Autodesk Fusion 360 part; units mm, degrees
note: some values were not read from the file. Chosen so that the rebuilt part matches the saved one: which bodies a step acts on.
(part 2 of 3)
sketch "DJ - Baxley - Dog Door (1)" plane through (0, 0, 0) normal (0, 1, 0) x (1, 0, 0)
  circle A0 through (-4.6949, -282.6663, -6.35) (-15.4673, -288.8858, -6.35) (-15.4673, -276.4469, -6.35)
  circle A1 through (-14.4863, -519.0473, -6.35) (-25.2588, -525.2667, -6.35) (-25.2588, -512.8278, -6.35)
  circle A2 through (-145.7196, -224.274, -6.35) (-156.4921, -230.4934, -6.35) (-156.4921, -218.0545, -6.35)
  circle A3 through (-70.3115, -135.2797, -6.35) (-81.084, -141.4992, -6.35) (-81.084, -129.0602, -6.35)
  circle A4 through (-80.103, -371.6606, -6.35) (-90.8754, -377.8801, -6.35) (-90.8754, -365.4411, -6.35)
  circle A5 through (60.9218, -430.053, -6.35) (50.1494, -436.2725, -6.35) (50.1494, -423.8335, -6.35)
  circle A6 through (51.1304, -666.4339, -6.35) (40.3579, -672.6534, -6.35) (40.3579, -660.2144, -6.35)
  circle A7 through (126.5385, -577.4396, -6.35) (115.766, -583.6591, -6.35) (115.766, -571.2202, -6.35)
  arc A8 through (0.0572, -283.1665, -6.35) (0.0572, -283.1665, -6.35) (0.0572, -283.1665, -6.35)
  arc A9 through (-65.5595, -135.7798, -6.35) (-65.5595, -135.7798, -6.35) (-65.5595, -135.7798, -6.35)
  arc A10 through (-9.7343, -519.5474, -6.35) (-9.7343, -519.5474, -6.35) (-9.7343, -519.5474, -6.35)
  arc A11 through (55.8824, -666.9341, -6.35) (55.8824, -666.9341, -6.35) (55.8824, -666.9341, -6.35)
  arc A12 through (65.6738, -430.5531, -6.35) (65.6738, -430.5531, -6.35) (65.6738, -430.5531, -6.35)
  arc A13 through (131.2905, -577.9398, -6.35) (131.2905, -577.9398, -6.35) (131.2905, -577.9398, -6.35)
  arc A14 through (-140.9676, -224.7741, -6.35) (-140.9676, -224.7741, -6.35) (-140.9676, -224.7741, -6.35)
  arc A15 through (-75.351, -372.1608, -6.35) (-75.351, -372.1608, -6.35) (-75.351, -372.1608, -6.35)
  circle A16 through (11.5572, -288.9047, -6.35) (0.7848, -295.1242, -6.35) (0.7848, -282.6852, -6.35)
  circle A17 through (1.7658, -525.2856, -6.35) (-9.0067, -531.5051, -6.35) (-9.0067, -519.0661, -6.35)
  circle A18 through (142.7906, -583.678, -6.35) (132.0181, -589.8975, -6.35) (132.0181, -577.4585, -6.35)
  circle A19 through (67.3825, -672.6723, -6.35) (56.61, -678.8917, -6.35) (56.61, -666.4528, -6.35)
  circle A20 through (77.1739, -436.2913, -6.35) (66.4015, -442.5108, -6.35) (66.4015, -430.0719, -6.35)
  circle A21 through (-129.4675, -230.5123, -6.35) (-140.24, -236.7318, -6.35) (-140.24, -224.2928, -6.35)
  circle A22 through (-54.0594, -141.518, -6.35) (-64.8319, -147.7375, -6.35) (-64.8319, -135.2986, -6.35)
  circle A23 through (-63.8509, -377.899, -6.35) (-74.6233, -384.1184, -6.35) (-74.6233, -371.6795, -6.35)
  circle A24 through (-46.9836, -370.3901, -6.35) (-57.756, -376.6096, -6.35) (-57.756, -364.1706, -6.35)
  circle A25 through (94.0412, -428.7825, -6.35) (83.2687, -435.0019, -6.35) (83.2687, -422.563, -6.35)
  circle A26 through (28.4245, -281.3958, -6.35) (17.6521, -287.6153, -6.35) (17.6521, -275.1763, -6.35)
  circle A27 through (84.2497, -665.1634, -6.35) (73.4773, -671.3829, -6.35) (73.4773, -658.9439, -6.35)
  circle A28 through (159.6579, -576.1691, -6.35) (148.8854, -582.3886, -6.35) (148.8854, -569.9496, -6.35)
  circle A29 through (18.6331, -517.7768, -6.35) (7.8606, -523.9962, -6.35) (7.8606, -511.5573, -6.35)
  circle A30 through (-37.1921, -134.0092, -6.35) (-47.9646, -140.2286, -6.35) (-47.9646, -127.7897, -6.35)
  circle A31 through (-112.6003, -223.0034, -6.35) (-123.3727, -229.2229, -6.35) (-123.3727, -216.784, -6.35)
  arc A32 through (11.5363, -288.3559, -6.35) (11.5363, -288.3559, -6.35) (11.5363, -288.3559, -6.35)
  arc A33 through (67.3615, -672.1235, -6.35) (67.3615, -672.1235, -6.35) (67.3615, -672.1235, -6.35)
  arc A34 through (77.1529, -435.7426, -6.35) (77.1529, -435.7426, -6.35) (77.1529, -435.7426, -6.35)
  arc A35 through (1.7448, -524.7369, -6.35) (1.7448, -524.7369, -6.35) (1.7448, -524.7369, -6.35)
  arc A36 through (142.7696, -583.1292, -6.35) (142.7696, -583.1292, -6.35) (142.7696, -583.1292, -6.35)
  arc A37 through (-63.8719, -377.3502, -6.35) (-63.8719, -377.3502, -6.35) (-63.8719, -377.3502, -6.35)
  arc A38 through (-129.4885, -229.9636, -6.35) (-129.4885, -229.9636, -6.35) (-129.4885, -229.9636, -6.35)
  arc A39 through (-54.0804, -140.9693, -6.35) (-54.0804, -140.9693, -6.35) (-54.0804, -140.9693, -6.35)
  circle A40 through (-40.7457, -354.1386, -6.35) (-51.5195, -360.3588, -6.35) (-51.5195, -347.9183, -6.35)
  circle A41 through (100.2791, -412.531, -6.35) (89.5053, -418.7512, -6.35) (89.5053, -406.3107, -6.35)
  circle A42 through (90.4876, -648.9119, -6.35) (79.7139, -655.1322, -6.35) (79.7139, -642.6916, -6.35)
  circle A43 through (34.6624, -265.1443, -6.35) (23.8886, -271.3646, -6.35) (23.8886, -258.9241, -6.35)
  circle A44 through (165.8958, -559.9176, -6.35) (155.122, -566.1379, -6.35) (155.122, -553.6974, -6.35)
  circle A45 through (24.871, -501.5252, -6.35) (14.0972, -507.7455, -6.35) (14.0972, -495.305, -6.35)
  circle A46 through (-106.3624, -206.7519, -6.35) (-117.1361, -212.9722, -6.35) (-117.1361, -200.5317, -6.35)
  circle A47 through (-30.9542, -117.7577, -6.35) (-41.728, -123.9779, -6.35) (-41.728, -111.5374, -6.35)
  arc A48 through (15.5928, -264.4328, -6.35) (15.6784, -265.1583, -6.35) (15.7364, -265.8867, -6.35)
  arc A49 through (51.9111, -657.7321, -6.35) (51.4996, -657.2579, -6.35) (51.0651, -656.8045, -6.35)
  arc A50 through (-11.9619, -270.2306, -6.35) (-17.8102, -266.2727, -6.35) (-19.7177, -259.4735, -6.35)
  arc A51 through (123.743, -544.5786, -6.35) (128.4893, -543.0332, -6.35) (132.5528, -540.1342, -6.35)
  arc A52 through (58.4262, -627.8801, -6.35) (72.1411, -628.2628, -6.35) (73.2112, -641.9413, -6.35)
  arc A53 through (71.5616, -649.6543, -6.35) (64.5815, -660.6144, -6.35) (51.9111, -657.7321, -6.35)
  arc A54 through (-4.7601, -273.037, -6.35) (-7.0021, -271.4358, -6.35) (-9.622, -270.5836, -6.35)
  arc A55 through (-59.6718, -354.8809, -6.35) (-66.6518, -365.8411, -6.35) (-79.3222, -362.9588, -6.35)
  arc A56 through (-95.1258, -348.4678, -6.35) (-92.29, -342.1526, -6.35) (-86.0885, -339.0761, -6.35)
  arc A57 through (-72.8072, -333.1068, -6.35) (-59.0922, -333.4895, -6.35) (-58.0221, -347.168, -6.35)
  arc A58 through (-17.2817, -486.1862, -6.35) (-12.5354, -484.6408, -6.35) (-8.472, -481.7418, -6.35)
  arc A59 through (120.553, -544.8551, -6.35) (122.1526, -544.7694, -6.35) (123.743, -544.5786, -6.35)
  arc A60 through (111.5156, -554.2468, -6.35) (114.3515, -547.9316, -6.35) (120.553, -544.8551, -6.35)
  arc A61 through (-79.3222, -362.9588, -6.35) (-79.7338, -362.4846, -6.35) (-80.1682, -362.0312, -6.35)
  arc A62 through (15.7364, -265.8867, -6.35) (8.7563, -276.8468, -6.35) (-3.9141, -273.9645, -6.35)
  arc A63 through (-19.7177, -259.4735, -6.35) (-16.8819, -253.1583, -6.35) (-10.6804, -250.0818, -6.35)
  arc A64 through (66.9361, -392.7476, -6.35) (67.5597, -392.1057, -6.35) (68.2176, -391.4992, -6.35)
  arc A65 through (-19.4134, -506.9645, -6.35) (-20.5908, -506.8371, -6.35) (-21.7533, -506.6116, -6.35)
  arc A66 through (45.899, -406.8602, -6.35) (48.7348, -400.545, -6.35) (54.9363, -397.4685, -6.35)
  arc A67 through (81.2094, -411.8194, -6.35) (81.2951, -412.545, -6.35) (81.353, -413.2733, -6.35)
  arc A68 through (-21.7533, -506.6116, -6.35) (-27.6017, -502.6537, -6.35) (-29.5091, -495.8545, -6.35)
  arc A69 through (5.8013, -500.8137, -6.35) (5.887, -501.5393, -6.35) (5.9449, -502.2676, -6.35)
  arc A70 through (81.353, -413.2733, -6.35) (74.373, -424.2335, -6.35) (61.7026, -421.3511, -6.35)
  arc A71 through (73.2112, -641.9413, -6.35) (71.7329, -644.9042, -6.35) (71.418, -648.2004, -6.35)
  arc A72 through (-85.0301, -359.5779, -6.35) (-86.2074, -359.4504, -6.35) (-87.37, -359.2249, -6.35)
  arc A73 through (146.9697, -560.66, -6.35) (139.9896, -571.6201, -6.35) (127.3193, -568.7378, -6.35)
  arc A74 through (-7.1905, -480.4935, -6.35) (6.5245, -480.8762, -6.35) (7.5945, -494.5547, -6.35)
  arc A75 through (146.8261, -559.2061, -6.35) (146.9118, -559.9317, -6.35) (146.9697, -560.66, -6.35)
  arc A76 through (17.386, -258.1737, -6.35) (15.9077, -261.1366, -6.35) (15.5928, -264.4328, -6.35)
  arc A77 through (-8.472, -481.7418, -6.35) (-7.8484, -481.1, -6.35) (-7.1905, -480.4935, -6.35)
  arc A78 through (36.1075, -643.2411, -6.35) (38.9434, -636.9259, -6.35) (45.1449, -633.8494, -6.35)
  arc A79 through (-82.8984, -338.7996, -6.35) (-78.1521, -337.2542, -6.35) (-74.0887, -334.3552, -6.35)
  arc A80 through (55.9947, -417.9702, -6.35) (54.8173, -417.8428, -6.35) (53.6548, -417.6173, -6.35)
  arc A81 through (60.8566, -420.4236, -6.35) (58.6146, -418.8224, -6.35) (55.9947, -417.9702, -6.35)
  arc A82 through (71.418, -648.2004, -6.35) (71.5036, -648.9259, -6.35) (71.5616, -649.6543, -6.35)
  arc A83 through (51.0651, -656.8045, -6.35) (48.8231, -655.2034, -6.35) (46.2032, -654.3512, -6.35)
  arc A84 through (133.8343, -538.8858, -6.35) (147.5492, -539.2685, -6.35) (148.6193, -552.9471, -6.35)
  arc A85 through (-80.1682, -362.0312, -6.35) (-82.4102, -360.4301, -6.35) (-85.0301, -359.5779, -6.35)
  arc A86 through (132.5528, -540.1342, -6.35) (133.1764, -539.4924, -6.35) (133.8343, -538.8858, -6.35)
  arc A87 through (-13.7055, -510.3454, -6.35) (-14.1171, -509.8712, -6.35) (-14.5516, -509.4179, -6.35)
  arc A88 through (-14.5516, -509.4179, -6.35) (-16.7935, -507.8167, -6.35) (-19.4134, -506.9645, -6.35)
  arc A89 through (-74.0887, -334.3552, -6.35) (-73.4651, -333.7134, -6.35) (-72.8072, -333.1068, -6.35)
  arc A90 through (53.6548, -417.6173, -6.35) (47.8064, -413.6594, -6.35) (45.899, -406.8602, -6.35)
  arc A91 through (61.7026, -421.3511, -6.35) (61.291, -420.8769, -6.35) (60.8566, -420.4236, -6.35)
  arc A92 through (-59.8154, -353.4271, -6.35) (-59.7297, -354.1526, -6.35) (-59.6718, -354.8809, -6.35)
  arc A93 through (83.0027, -405.5604, -6.35) (81.5244, -408.5233, -6.35) (81.2094, -411.8194, -6.35)
  arc A94 through (43.8633, -653.9982, -6.35) (38.015, -650.0403, -6.35) (36.1075, -643.2411, -6.35)
  arc A95 through (68.2176, -391.4992, -6.35) (81.9326, -391.8819, -6.35) (83.0027, -405.5604, -6.35)
  arc A96 through (-29.5091, -495.8545, -6.35) (-26.6733, -489.5393, -6.35) (-20.4718, -486.4628, -6.35)
  arc A97 through (121.6114, -565.3569, -6.35) (120.434, -565.2294, -6.35) (119.2714, -565.0039, -6.35)
  arc A98 through (126.4732, -567.8103, -6.35) (124.2313, -566.2091, -6.35) (121.6114, -565.3569, -6.35)
  arc A99 through (-9.622, -270.5836, -6.35) (-10.7993, -270.4561, -6.35) (-11.9619, -270.2306, -6.35)
  arc A100 through (45.1449, -633.8494, -6.35) (46.7444, -633.7637, -6.35) (48.3349, -633.5729, -6.35)
  arc A101 through (148.6193, -552.9471, -6.35) (147.1411, -555.9099, -6.35) (146.8261, -559.2061, -6.35)
  arc A102 through (-7.4903, -249.8053, -6.35) (-2.744, -248.2599, -6.35) (1.3195, -245.3609, -6.35)
  arc A103 through (58.1264, -397.1919, -6.35) (62.8727, -395.6465, -6.35) (66.9361, -392.7476, -6.35)
  arc A104 through (48.3349, -633.5729, -6.35) (53.0812, -632.0275, -6.35) (57.1447, -629.1285, -6.35)
  arc A105 through (119.2714, -565.0039, -6.35) (113.4231, -561.0461, -6.35) (111.5156, -554.2468, -6.35)
  arc A106 through (7.5945, -494.5547, -6.35) (6.1163, -497.5176, -6.35) (5.8013, -500.8137, -6.35)
  arc A107 through (-20.4718, -486.4628, -6.35) (-18.8722, -486.377, -6.35) (-17.2817, -486.1862, -6.35)
  arc A108 through (-87.37, -359.2249, -6.35) (-93.2184, -355.267, -6.35) (-95.1258, -348.4678, -6.35)
  arc A109 through (-49.8803, -118.5, -6.35) (-56.8604, -129.4602, -6.35) (-69.5307, -126.5778, -6.35)
  arc A110 through (-150.6468, -212.1912, -6.35) (-151.8241, -212.0638, -6.35) (-152.9867, -211.8383, -6.35)
  arc A111 through (-85.3344, -112.0869, -6.35) (-82.4985, -105.7717, -6.35) (-76.297, -102.6952, -6.35)
  arc A112 through (1.3195, -245.3609, -6.35) (1.943, -244.7191, -6.35) (2.6009, -244.1125, -6.35)
  arc A113 through (-10.6804, -250.0818, -6.35) (-9.0808, -249.9961, -6.35) (-7.4903, -249.8053, -6.35)
  arc A114 through (-152.9867, -211.8383, -6.35) (-158.835, -207.8804, -6.35) (-160.7425, -201.0812, -6.35)
  arc A115 through (2.6009, -244.1125, -6.35) (16.3159, -244.4952, -6.35) (17.386, -258.1737, -6.35)
  arc A116 through (-160.7425, -201.0812, -6.35) (-157.9066, -194.766, -6.35) (-151.7051, -191.6894, -6.35)
  arc A117 through (54.9363, -397.4685, -6.35) (56.5359, -397.3827, -6.35) (58.1264, -397.1919, -6.35)
  arc A118 through (-64.2972, -97.9742, -6.35) (-63.6736, -97.3324, -6.35) (-63.0157, -96.7259, -6.35)
  arc A119 through (-63.0157, -96.7259, -6.35) (-49.3008, -97.1086, -6.35) (-48.2307, -110.7871, -6.35)
  arc A120 through (-77.5786, -122.844, -6.35) (-83.4269, -118.8861, -6.35) (-85.3344, -112.0869, -6.35)
  arc A121 through (5.9449, -502.2676, -6.35) (-1.0352, -513.2278, -6.35) (-13.7055, -510.3454, -6.35)
  arc A122 through (-151.7051, -191.6894, -6.35) (-150.1056, -191.6037, -6.35) (-148.5151, -191.4129, -6.35)
  arc A123 through (-69.5307, -126.5778, -6.35) (-69.9423, -126.1036, -6.35) (-70.3768, -125.6503, -6.35)
  arc A124 through (-125.2884, -207.4943, -6.35) (-132.2685, -218.4544, -6.35) (-144.9389, -215.5721, -6.35)
  arc A125 through (-125.432, -206.0404, -6.35) (-125.3464, -206.766, -6.35) (-125.2884, -207.4943, -6.35)
  arc A126 through (-73.107, -102.4186, -6.35) (-68.3607, -100.8732, -6.35) (-64.2972, -97.9742, -6.35)
  arc A127 through (-139.7053, -186.9685, -6.35) (-139.0818, -186.3267, -6.35) (-138.4238, -185.7202, -6.35)
  arc A128 through (127.3193, -568.7378, -6.35) (126.9077, -568.2636, -6.35) (126.4732, -567.8103, -6.35)
  arc A129 through (-58.0221, -347.168, -6.35) (-59.5004, -350.1309, -6.35) (-59.8154, -353.4271, -6.35)
  arc A130 through (-138.4238, -185.7202, -6.35) (-124.7089, -186.1029, -6.35) (-123.6388, -199.7814, -6.35)
  arc A131 through (-123.6388, -199.7814, -6.35) (-125.1171, -202.7443, -6.35) (-125.432, -206.0404, -6.35)
  arc A132 through (-145.7849, -214.6446, -6.35) (-148.0269, -213.0434, -6.35) (-150.6468, -212.1912, -6.35)
  arc A133 through (-148.5151, -191.4129, -6.35) (-143.7688, -189.8675, -6.35) (-139.7053, -186.9685, -6.35)
  arc A134 through (-86.0885, -339.0761, -6.35) (-84.4889, -338.9904, -6.35) (-82.8984, -338.7996, -6.35)
  arc A135 through (-144.9389, -215.5721, -6.35) (-145.3504, -215.0979, -6.35) (-145.7849, -214.6446, -6.35)
  arc A136 through (-48.2307, -110.7871, -6.35) (-49.7089, -113.75, -6.35) (-50.0239, -117.0461, -6.35)
  arc A137 through (-75.2386, -123.1969, -6.35) (-76.416, -123.0695, -6.35) (-77.5786, -122.844, -6.35)
  arc A138 through (57.1447, -629.1285, -6.35) (57.7682, -628.4867, -6.35) (58.4262, -627.8801, -6.35)
  arc A139 through (-50.0239, -117.0461, -6.35) (-49.9382, -117.7717, -6.35) (-49.8803, -118.5, -6.35)
  arc A140 through (-76.297, -102.6952, -6.35) (-74.6974, -102.6094, -6.35) (-73.107, -102.4186, -6.35)
  arc A141 through (46.2032, -654.3512, -6.35) (45.0259, -654.2237, -6.35) (43.8633, -653.9982, -6.35)
  arc A142 through (-3.9141, -273.9645, -6.35) (-4.3257, -273.4903, -6.35) (-4.7601, -273.037, -6.35)
  arc A143 through (-70.3768, -125.6503, -6.35) (-72.6187, -124.0491, -6.35) (-75.2386, -123.1969, -6.35)
  arc A144 through (89.7833, -401.0546, -6.35) (104.3795, -408.6094, -6.35) (97.6152, -423.5883, -6.35)
  arc A145 through (37.6424, -656.2906, -6.35) (32.7318, -650.409, -6.35) (31.3594, -642.8709, -6.35)
  arc A146 through (15.8916, -292.0741, -6.35) (5.0873, -300.8276, -6.35) (-6.6815, -293.4215, -6.35)
  arc A147 through (122.9961, -539.8749, -6.35) (126.3046, -538.8011, -6.35) (129.1496, -536.7999, -6.35)
  arc A148 through (129.1496, -536.7999, -6.35) (129.9179, -536.0182, -6.35) (130.7258, -535.2775, -6.35)
  arc A149 through (79.9919, -637.4356, -6.35) (94.5881, -644.9904, -6.35) (87.8237, -659.9693, -6.35)
  arc A150 through (54.6438, -392.71, -6.35) (56.0155, -392.6472, -6.35) (57.3795, -392.4883, -6.35)
  arc A151 through (120.2605, -540.0967, -6.35) (121.6322, -540.0338, -6.35) (122.9961, -539.8749, -6.35)
  arc A152 through (-27.9743, -508.904, -6.35) (-32.8849, -503.0224, -6.35) (-34.2572, -495.4843, -6.35)
  arc A153 through (6.1001, -528.455, -6.35) (-4.7041, -537.2085, -6.35) (-16.473, -529.8025, -6.35)
  arc A154 through (97.6152, -423.5883, -6.35) (95.2432, -437.29, -6.35) (81.5082, -439.4607, -6.35)
  arc A155 through (-18.0287, -481.4826, -6.35) (-14.7202, -480.4087, -6.35) (-11.8752, -478.4075, -6.35)
  arc A156 through (31.3594, -642.8709, -6.35) (35.6027, -633.5299, -6.35) (44.8524, -629.091, -6.35)
  arc A157 through (44.8524, -629.091, -6.35) (46.2241, -629.0281, -6.35) (47.588, -628.8692, -6.35)
  arc A158 through (106.7676, -553.8766, -6.35) (111.0108, -544.5356, -6.35) (120.2605, -540.0967, -6.35)
  arc A159 through (55.3177, -624.2718, -6.35) (72.1418, -622.4433, -6.35) (79.9919, -637.4356, -6.35)
  arc A160 through (147.1249, -586.8474, -6.35) (136.3207, -595.6009, -6.35) (124.5518, -588.1948, -6.35)
  arc A161 through (113.0505, -567.2963, -6.35) (108.1399, -561.4147, -6.35) (106.7676, -553.8766, -6.35)
  arc A162 through (71.7168, -675.8417, -6.35) (60.9125, -684.5952, -6.35) (49.1437, -677.1891, -6.35)
  arc A163 through (87.8237, -659.9693, -6.35) (85.4517, -673.6709, -6.35) (71.7168, -675.8417, -6.35)
  arc A164 through (130.7258, -535.2775, -6.35) (147.5499, -533.449, -6.35) (155.4, -548.4413, -6.35)
  arc A165 through (47.588, -628.8692, -6.35) (50.8964, -627.7953, -6.35) (53.7415, -625.7942, -6.35)
  arc A166 through (124.5518, -588.1948, -6.35) (108.8928, -583.1986, -6.35) (113.0505, -567.2963, -6.35)
  arc A167 through (53.7415, -625.7942, -6.35) (54.5098, -625.0125, -6.35) (55.3177, -624.2718, -6.35)
  arc A168 through (49.1437, -677.1891, -6.35) (33.4847, -672.1929, -6.35) (37.6424, -656.2906, -6.35)
  arc A169 through (-67.7004, -94.64, -6.35) (-66.9321, -93.8582, -6.35) (-66.1242, -93.1176, -6.35)
  arc A170 through (155.4, -548.4413, -6.35) (169.9962, -555.9961, -6.35) (163.2319, -570.975, -6.35)
  arc A171 through (-33.6181, -128.815, -6.35) (-35.9902, -142.5167, -6.35) (-49.7251, -144.6874, -6.35)
  arc A172 through (163.2319, -570.975, -6.35) (160.8598, -584.6766, -6.35) (147.1249, -586.8474, -6.35)
  arc A173 through (-77.4918, -331.0209, -6.35) (-76.7236, -330.2392, -6.35) (-75.9156, -329.4985, -6.35)
  arc A174 through (-151.9976, -186.931, -6.35) (-150.6259, -186.8682, -6.35) (-149.262, -186.7093, -6.35)
  arc A175 through (-51.2415, -342.6623, -6.35) (-36.6453, -350.2171, -6.35) (-43.4096, -365.196, -6.35)
  arc A176 through (-24.4658, -259.1033, -6.35) (-20.2225, -249.7623, -6.35) (-10.9728, -245.3234, -6.35)
  arc A177 through (-8.2372, -245.1016, -6.35) (-4.9288, -244.0277, -6.35) (-2.0837, -242.0266, -6.35)
  arc A178 through (-147.7063, -235.0292, -6.35) (-163.3653, -230.0329, -6.35) (-159.2076, -214.1306, -6.35)
  arc A179 through (-83.6453, -334.0959, -6.35) (-80.3369, -333.022, -6.35) (-77.4918, -331.0209, -6.35)
  arc A180 through (-75.9156, -329.4985, -6.35) (-59.0916, -327.67, -6.35) (-51.2415, -342.6623, -6.35)
  arc A181 through (-99.8739, -348.0976, -6.35) (-95.6306, -338.7566, -6.35) (-86.3809, -334.3177, -6.35)
  arc A182 through (-59.5166, -381.0684, -6.35) (-70.3208, -389.8219, -6.35) (-82.0896, -382.4158, -6.35)
  arc A183 through (-43.4096, -365.196, -6.35) (-45.7816, -378.8976, -6.35) (-59.5166, -381.0684, -6.35)
  arc A184 through (-82.0896, -382.4158, -6.35) (-97.7487, -377.4196, -6.35) (-93.591, -361.5173, -6.35)
  arc A185 through (-76.5895, -97.9367, -6.35) (-75.2178, -97.8739, -6.35) (-73.8539, -97.715, -6.35)
  arc A186 through (-125.1332, -233.6817, -6.35) (-135.9375, -242.4352, -6.35) (-147.7063, -235.0292, -6.35)
  arc A187 through (-86.3809, -334.3177, -6.35) (-85.0092, -334.2548, -6.35) (-83.6453, -334.0959, -6.35)
  arc A188 through (-2.0837, -242.0266, -6.35) (-1.3154, -241.2449, -6.35) (-0.5075, -240.5042, -6.35)
  arc A189 through (-73.8539, -97.715, -6.35) (-70.5454, -96.6411, -6.35) (-67.7004, -94.64, -6.35)
  arc A190 through (-93.591, -361.5173, -6.35) (-98.5015, -355.6357, -6.35) (-99.8739, -348.0976, -6.35)
  arc A191 through (24.1667, -253.668, -6.35) (38.7629, -261.2228, -6.35) (31.9985, -276.2017, -6.35)
  arc A192 through (-41.45, -106.2813, -6.35) (-26.8538, -113.8361, -6.35) (-33.6181, -128.815, -6.35)
  arc A193 through (-18.1828, -272.523, -6.35) (-23.0934, -266.6414, -6.35) (-24.4658, -259.1033, -6.35)
  arc A194 through (-66.1242, -93.1176, -6.35) (-49.3001, -91.2891, -6.35) (-41.45, -106.2813, -6.35)
  arc A195 through (-49.7251, -144.6874, -6.35) (-60.5293, -153.4409, -6.35) (-72.2982, -146.0349, -6.35)
  arc A196 through (-10.9728, -245.3234, -6.35) (-9.6011, -245.2605, -6.35) (-8.2372, -245.1016, -6.35)
  arc A197 through (-72.2982, -146.0349, -6.35) (-87.9572, -141.0386, -6.35) (-83.7995, -125.1364, -6.35)
  arc A198 through (-109.0263, -217.8093, -6.35) (-111.3983, -231.5109, -6.35) (-125.1332, -233.6817, -6.35)
  arc A199 through (-20.7643, -481.7043, -6.35) (-19.3926, -481.6415, -6.35) (-18.0287, -481.4826, -6.35)
  arc A200 through (14.3752, -490.0489, -6.35) (28.9714, -497.6037, -6.35) (22.2071, -512.5826, -6.35)
  arc A201 through (-149.262, -186.7093, -6.35) (-145.9536, -185.6354, -6.35) (-143.1085, -183.6342, -6.35)
  arc A202 through (58.9352, -440.8082, -6.35) (43.2761, -435.8119, -6.35) (47.4338, -419.9097, -6.35)
  arc A203 through (63.533, -389.4133, -6.35) (64.3012, -388.6315, -6.35) (65.1092, -387.8909, -6.35)
  arc A204 through (81.5082, -439.4607, -6.35) (70.704, -448.2142, -6.35) (58.9352, -440.8082, -6.35)
  arc A205 through (-143.1085, -183.6342, -6.35) (-142.3402, -182.8525, -6.35) (-141.5323, -182.1119, -6.35)
  arc A206 through (-165.4906, -200.711, -6.35) (-161.2473, -191.3699, -6.35) (-151.9976, -186.931, -6.35)
  arc A207 through (31.9985, -276.2017, -6.35) (29.6265, -289.9033, -6.35) (15.8916, -292.0741, -6.35)
  arc A208 through (65.1092, -387.8909, -6.35) (81.9332, -386.0624, -6.35) (89.7833, -401.0546, -6.35)
  arc A209 through (57.3795, -392.4883, -6.35) (60.6879, -391.4144, -6.35) (63.533, -389.4133, -6.35)
  arc A210 through (22.2071, -512.5826, -6.35) (19.835, -526.2842, -6.35) (6.1001, -528.455, -6.35)
  arc A211 through (-0.5075, -240.5042, -6.35) (16.3166, -238.6757, -6.35) (24.1667, -253.668, -6.35)
  arc A212 through (-34.2572, -495.4843, -6.35) (-30.014, -486.1432, -6.35) (-20.7643, -481.7043, -6.35)
  arc A213 through (41.1509, -406.49, -6.35) (45.3942, -397.1489, -6.35) (54.6438, -392.71, -6.35)
  arc A214 through (-6.6815, -293.4215, -6.35) (-22.3406, -288.4253, -6.35) (-18.1828, -272.523, -6.35)
  arc A215 through (-11.8752, -478.4075, -6.35) (-11.1069, -477.6258, -6.35) (-10.2989, -476.8852, -6.35)
  arc A216 through (-159.2076, -214.1306, -6.35) (-164.1182, -208.2491, -6.35) (-165.4906, -200.711, -6.35)
  arc A217 through (-116.8581, -195.2756, -6.35) (-102.2619, -202.8304, -6.35) (-109.0263, -217.8093, -6.35)
  arc A218 through (-10.2989, -476.8852, -6.35) (6.5251, -475.0567, -6.35) (14.3752, -490.0489, -6.35)
  arc A219 through (-16.473, -529.8025, -6.35) (-32.132, -524.8062, -6.35) (-27.9743, -508.904, -6.35)
  arc A220 through (47.4338, -419.9097, -6.35) (42.5233, -414.0281, -6.35) (41.1509, -406.49, -6.35)
  arc A221 through (-141.5323, -182.1119, -6.35) (-124.7082, -180.2834, -6.35) (-116.8581, -195.2756, -6.35)
  arc A222 through (-90.0824, -111.7167, -6.35) (-85.8392, -102.3756, -6.35) (-76.5895, -97.9367, -6.35)
  arc A223 through (-83.7995, -125.1364, -6.35) (-88.7101, -119.2548, -6.35) (-90.0824, -111.7167, -6.35)
  line L0 (-266.5509, -596.9, -6.35) -> (-266.5509, 0, -6.35)
  arc A224 through (266.8491, -596.9, -6.35) (0.1491, -863.6, -6.35) (-266.5509, -596.9, -6.35)
  line L1 (266.8491, 0, -6.35) -> (266.8491, -596.9, -6.35)
  line L2 (241.4491, 0, -6.35) -> (266.8491, 0, -6.35)
  line L3 (-241.1509, 0, -6.35) -> (-241.1509, -411.8539, -6.35)
  arc A225 through (-241.1509, -596.9, -6.35) (0.1491, -838.2, -6.35) (241.4491, -596.9, -6.35)
  line L4 (-241.1509, -439.1647, -6.35) -> (-241.1509, -596.9, -6.35)
  line L5 (241.4491, -596.9, -6.35) -> (241.4491, 0, -6.35)
  line L6 (-215.7509, -25.4, -6.35) -> (-215.7509, -420.1147, -6.35)
  arc A226 through (-215.7509, -596.9, -6.35) (0.1491, -812.8, -6.35) (216.0491, -596.9, -6.35)
  line L7 (216.0491, -596.9, -6.35) -> (216.0491, -25.4, -6.35)
  line L8 (-215.7509, -439.1647, -6.35) -> (-215.7509, -596.9, -6.35)
  line L9 (-190.3509, -50.8, -6.35) -> (-190.3509, -420.1147, -6.35)
  line L10 (190.6491, -596.9, -6.35) -> (190.6491, -50.8, -6.35)
  line L11 (-190.3509, -439.1647, -6.35) -> (-190.3509, -596.9, -6.35)
  arc A227 through (-190.3509, -596.9, -6.35) (0.1491, -787.4, -6.35) (190.6491, -596.9, -6.35)
  line L12 (216.0491, -25.4, -6.35) -> (-215.7509, -25.4, -6.35)
  line L13 (190.6491, -50.8, -6.35) -> (-190.3509, -50.8, -6.35)
  circle A228 through (-196.7009, -429.6397, -6.35) (-206.2259, -435.139, -6.35) (-206.2259, -424.1405, -6.35)
  line L14 (-260.2009, -411.8539, -6.35) -> (-241.1509, -411.8539, -6.35)
  line L15 (-241.1509, -411.8539, -6.35) -> (-241.1509, -428.0522, -6.35)
  line L16 (-241.1509, -428.0522, -6.35) -> (-260.2009, -428.0522, -6.35)
  line L17 (-260.2009, -428.0522, -6.35) -> (-260.2009, -411.8539, -6.35)
  arc A229 through (-152.1305, -436.5446, -6.35) (-150.9878, -436.3044, -6.35) (-151.004, -435.1368, -6.35)
  line L18 (-261.7725, -439.1647, -6.35) -> (-186.7302, -439.1647, -6.35)
  arc A230 through (-184.4429, -438.341, -6.35) (-168.61, -431.6265, -6.35) (-152.1305, -436.5446, -6.35)
  line L19 (-260.2009, -420.1147, -6.35) -> (-261.7725, -420.1147, -6.35)
  line L20 (-181.8374, -420.1147, -6.35) -> (-241.1509, -420.1147, -6.35)
  arc A231 through (-151.004, -435.1368, -6.35) (-164.5769, -423.8412, -6.35) (-181.8374, -420.1147, -6.35)
  arc A232 through (-261.7725, -420.1147, -6.35) (-263.4987, -429.6397, -6.35) (-261.7725, -439.1647, -6.35)
  arc A233 through (-186.7302, -439.1647, -6.35) (-185.5151, -438.9513, -6.35) (-184.4429, -438.341, -6.35)
  line L21 (222.3991, -25.4, -6.35) -> (235.0991, -25.4, -6.35)
  line L22 (235.0991, -25.4, -6.35) -> (235.0991, -101.6, -6.35)
  line L23 (235.0991, -101.6, -6.35) -> (222.3991, -101.6, -6.35)
  line L24 (222.3991, -101.6, -6.35) -> (222.3991, -25.4, -6.35)
  line L25 (222.3991, -63.5, -6.35) -> (235.0991, -63.5, -6.35)
  line L26 (216.0491, -25.4, -6.35) -> (216.0491, -63.5, -6.35)
  line L27 (216.0491, -63.5, -6.35) -> (222.3991, -63.5, -6.35)
  line L28 (222.3991, -63.5, -6.35) -> (222.3991, -25.4, -6.35)
  line L29 (222.3991, -25.4, -6.35) -> (216.0491, -25.4, -6.35)
  line L30 (235.0991, -101.6, -6.35) -> (241.4491, -101.6, -6.35)
  line L31 (235.0991, -63.5, -6.35) -> (235.0991, -101.6, -6.35)
  line L32 (241.4491, -63.5, -6.35) -> (235.0991, -63.5, -6.35)
  line L33 (241.4491, -101.6, -6.35) -> (241.4491, -63.5, -6.35)
  line L34 (222.3991, -518.7254, -6.35) -> (235.0991, -518.7254, -6.35)
  line L35 (235.0991, -594.9254, -6.35) -> (222.3991, -594.9254, -6.35)
  line L36 (222.3991, -594.9254, -6.35) -> (222.3991, -518.7254, -6.35)
  line L37 (235.0991, -518.7254, -6.35) -> (235.0991, -594.9254, -6.35)
  line L38 (222.3991, -556.8254, -6.35) -> (235.0991, -556.8254, -6.35)
  line L39 (216.0491, -518.7254, -6.35) -> (216.0491, -556.8254, -6.35)
  line L40 (222.3991, -556.8254, -6.35) -> (222.3991, -518.7254, -6.35)
  line L41 (222.3991, -518.7254, -6.35) -> (216.0491, -518.7254, -6.35)
  line L42 (216.0491, -556.8254, -6.35) -> (222.3991, -556.8254, -6.35)
  line L43 (241.4491, -556.8254, -6.35) -> (235.0991, -556.8254, -6.35)
  line L44 (235.0991, -556.8254, -6.35) -> (235.0991, -594.9254, -6.35)
  line L45 (235.0991, -594.9254, -6.35) -> (241.4491, -594.9254, -6.35)
  line L46 (241.4491, -594.9254, -6.35) -> (241.4491, -556.8254, -6.35)
  line L47 (6.4991, -50.8, -6.35) -> (6.4991, -237.1607, -6.35)
  line L48 (6.4991, -242.0445, -6.35) -> (6.4991, -277.5095, -6.35)
  line L49 (6.4991, -282.0442, -6.35) -> (6.4991, -295.7652, -6.35)
  line L50 (6.4991, -300.6585, -6.35) -> (6.4991, -475.0428, -6.35)
  line L51 (6.4991, -480.8522, -6.35) -> (6.4991, -496.4423, -6.35)
  line L52 (6.4991, -512.5757, -6.35) -> (6.4991, -522.9778, -6.35)
  line L53 (6.4991, -528.6458, -6.35) -> (6.4991, -787.2941, -6.35)
  line L54 (-6.2009, -50.8, -6.35) -> (-6.2009, -244.5718, -6.35)
  line L55 (-6.2009, -249.5407, -6.35) -> (-6.2009, -272.1568, -6.35)
  line L56 (-6.2009, -278.266, -6.35) -> (-6.2009, -287.0667, -6.35)
  line L57 (-6.2009, -294.4545, -6.35) -> (-6.2009, -474.3935, -6.35)
  line L58 (-6.2009, -479.7502, -6.35) -> (-6.2009, -514.0409, -6.35)
  line L59 (-6.2009, -518.147, -6.35) -> (-6.2009, -532.4242, -6.35)
  line L60 (-6.2009, -537.2039, -6.35) -> (-6.2009, -787.2941, -6.35)
  line L61 (-59.1175, -50.8, -6.35) -> (-59.1175, -89.7741, -6.35)
  line L62 (-59.1175, -94.6578, -6.35) -> (-59.1175, -130.1228, -6.35)
  line L63 (-59.1175, -134.6575, -6.35) -> (-59.1175, -148.3785, -6.35)
  line L64 (-59.1175, -153.2719, -6.35) -> (-59.1175, -327.6562, -6.35)
  line L65 (-59.1175, -333.4655, -6.35) -> (-59.1175, -349.0556, -6.35)
  line L66 (-59.1175, -365.1891, -6.35) -> (-59.1175, -375.5911, -6.35)
  line L67 (-59.1175, -381.2592, -6.35) -> (-59.1175, -777.9462, -6.35)
  line L68 (-71.8175, -50.8, -6.35) -> (-71.8175, -97.1851, -6.35)
  line L69 (-71.8175, -102.1541, -6.35) -> (-71.8175, -124.5061, -6.35)
  line L70 (-71.8175, -130.8793, -6.35) -> (-71.8175, -139.68, -6.35)
  line L71 (-71.8175, -147.0678, -6.35) -> (-71.8175, -327.0069, -6.35)
  line L72 (-71.8175, -332.3636, -6.35) -> (-71.8175, -366.6542, -6.35)
  line L73 (-71.8175, -370.7604, -6.35) -> (-71.8175, -385.0376, -6.35)
  line L74 (-71.8175, -389.8173, -6.35) -> (-71.8175, -773.2832, -6.35)
  line L75 (72.1158, -50.8, -6.35) -> (72.1158, -384.5474, -6.35)
  line L76 (72.1158, -389.4311, -6.35) -> (72.1158, -424.8962, -6.35)
  line L77 (72.1158, -429.4308, -6.35) -> (72.1158, -443.1518, -6.35)
  line L78 (72.1158, -448.0452, -6.35) -> (72.1158, -622.4295, -6.35)
  line L79 (72.1158, -628.2388, -6.35) -> (72.1158, -643.8289, -6.35)
  line L80 (72.1158, -659.9624, -6.35) -> (72.1158, -670.3644, -6.35)
  line L81 (72.1158, -676.0325, -6.35) -> (72.1158, -773.2832, -6.35)
  line L82 (59.4158, -50.8, -6.35) -> (59.4158, -391.9584, -6.35)
  line L83 (59.4158, -396.9274, -6.35) -> (59.4158, -419.5435, -6.35)
  line L84 (59.4158, -425.6526, -6.35) -> (59.4158, -434.4533, -6.35)
  line L85 (59.4158, -441.8411, -6.35) -> (59.4158, -621.7802, -6.35)
  line L86 (59.4158, -627.1369, -6.35) -> (59.4158, -661.4275, -6.35)
  line L87 (59.4158, -665.5337, -6.35) -> (59.4158, -679.8109, -6.35)
  line L88 (59.4158, -684.5906, -6.35) -> (59.4158, -777.9462, -6.35)
  line L89 (137.7325, -50.8, -6.35) -> (137.7325, -531.934, -6.35)
  line L90 (137.7325, -536.8178, -6.35) -> (137.7325, -572.2828, -6.35)
  line L91 (137.7325, -576.8175, -6.35) -> (137.7325, -590.5385, -6.35)
  line L92 (137.7325, -595.4318, -6.35) -> (137.7325, -728.6614, -6.35)
  line L93 (125.0325, -50.8, -6.35) -> (125.0325, -539.3451, -6.35)
  line L94 (125.0325, -544.314, -6.35) -> (125.0325, -566.6661, -6.35)
  line L95 (125.0325, -573.0393, -6.35) -> (125.0325, -581.84, -6.35)
  line L96 (125.0325, -589.2278, -6.35) -> (125.0325, -740.7555, -6.35)
  line L97 (-124.7342, -50.8, -6.35) -> (-124.7342, -180.2695, -6.35)
  line L98 (-124.7342, -186.0789, -6.35) -> (-124.7342, -201.669, -6.35)
  line L99 (-124.7342, -217.8024, -6.35) -> (-124.7342, -228.2045, -6.35)
  line L100 (-124.7342, -233.8725, -6.35) -> (-124.7342, -740.7555, -6.35)
  line L101 (-137.4342, -50.8, -6.35) -> (-137.4342, -179.6202, -6.35)
  line L102 (-137.4342, -184.9769, -6.35) -> (-137.4342, -219.2676, -6.35)
  line L103 (-137.4342, -223.3737, -6.35) -> (-137.4342, -237.6509, -6.35)
  line L104 (-137.4342, -242.4306, -6.35) -> (-137.4342, -728.6614, -6.35)
  line L105 (284.6029, 0, -6.35) -> (-289.1743, 0, -6.35)
sketch "DJ - Baxley - Dog Door (1) (curves -6.35 mm off its plane)" plane through (0, -6.35, 0) normal (0, 1, 0) x (1, 0, 0)
  circle A0 centre (-11.8765, -282.6663) radius 7.1816
  circle A1 centre (-21.6679, -519.0473) radius 7.1816
  circle A2 centre (-152.9013, -224.274) radius 7.1816
  circle A3 centre (-77.4932, -135.2797) radius 7.1816
  circle A4 centre (-87.2846, -371.6606) radius 7.1816
  circle A5 centre (53.7402, -430.053) radius 7.1816
  circle A6 centre (43.9487, -666.4339) radius 7.1816
  circle A7 centre (119.3568, -577.4396) radius 7.1816
  arc A8 (0.0572, -283.1665) -> (0.0572, -283.1665) centre (-11.8765, -282.6663) cw
  arc A9 (-65.5595, -135.7798) -> (-65.5595, -135.7798) centre (-77.4932, -135.2797) cw
  arc A10 (-9.7343, -519.5474) -> (-9.7343, -519.5474) centre (-21.6679, -519.0473) cw
  arc A11 (55.8824, -666.9341) -> (55.8824, -666.9341) centre (43.9487, -666.4339) cw
  arc A12 (65.6738, -430.5531) -> (65.6738, -430.5531) centre (53.7402, -430.053) cw
  arc A13 (131.2905, -577.9398) -> (131.2905, -577.9398) centre (119.3568, -577.4396) cw
  arc A14 (-140.9676, -224.7741) -> (-140.9676, -224.7741) centre (-152.9013, -224.274) cw
  arc A15 (-75.351, -372.1608) -> (-75.351, -372.1608) centre (-87.2846, -371.6606) cw
  circle A16 centre (4.3756, -288.9047) radius 7.1816
  circle A17 centre (-5.4158, -525.2856) radius 7.1816
  circle A18 centre (135.609, -583.678) radius 7.1816
  circle A19 centre (60.2008, -672.6723) radius 7.1816
  circle A20 centre (69.9923, -436.2913) radius 7.1816
  circle A21 centre (-136.6492, -230.5123) radius 7.1816
  circle A22 centre (-61.241, -141.518) radius 7.1816
  circle A23 centre (-71.0325, -377.899) radius 7.1816
  circle A24 centre (-54.1652, -370.3901) radius 7.1816
  circle A25 centre (86.8596, -428.7825) radius 7.1816
  circle A26 centre (21.2429, -281.3958) radius 7.1816
  circle A27 centre (77.0681, -665.1634) radius 7.1816
  circle A28 centre (152.4762, -576.1691) radius 7.1816
  circle A29 centre (11.4514, -517.7768) radius 7.1816
  circle A30 centre (-44.3738, -134.0092) radius 7.1816
  circle A31 centre (-119.7819, -223.0034) radius 7.1816
  arc A32 (11.5363, -288.3559) -> (11.5363, -288.3559) centre (21.2429, -281.3958) cw
  arc A33 (67.3615, -672.1235) -> (67.3615, -672.1235) centre (77.0681, -665.1634) cw
  arc A34 (77.1529, -435.7426) -> (77.1529, -435.7426) centre (86.8596, -428.7825) cw
  arc A35 (1.7448, -524.7369) -> (1.7448, -524.7369) centre (11.4514, -517.7768) cw
  arc A36 (142.7696, -583.1292) -> (142.7696, -583.1292) centre (152.4762, -576.1691) cw
  arc A37 (-63.8719, -377.3502) -> (-63.8719, -377.3502) centre (-54.1652, -370.3901) cw
  arc A38 (-129.4885, -229.9636) -> (-129.4885, -229.9636) centre (-119.7819, -223.0034) cw
  arc A39 (-54.0804, -140.9693) -> (-54.0804, -140.9693) centre (-44.3738, -134.0092) cw
  circle A40 centre (-47.9282, -354.1386) radius 7.1825
  circle A41 centre (93.0966, -412.531) radius 7.1825
  circle A42 centre (83.3051, -648.9119) radius 7.1825
  circle A43 centre (27.4799, -265.1443) radius 7.1825
  circle A44 centre (158.7132, -559.9176) radius 7.1825
  circle A45 centre (17.6884, -501.5252) radius 7.1825
  circle A46 centre (-113.5449, -206.7519) radius 7.1825
  circle A47 centre (-38.1368, -117.7577) radius 7.1825
  arc A48 (15.5928, -264.4328) -> (15.7364, -265.8867) centre (-3.3884, -267.0415) cw
  arc A49 (51.9111, -657.7321) -> (51.0651, -656.8045) centre (42.0867, -665.8437) ccw
  arc A50 (-11.9619, -270.2306) -> (-19.7177, -259.4735) centre (-9.4843, -260.2698) cw
  arc A51 (123.743, -544.5786) -> (132.5528, -540.1342) centre (121.087, -528.3601) ccw
  arc A52 (58.4262, -627.8801) -> (73.2112, -641.9413) centre (65.0709, -635.6971) cw
  arc A53 (71.5616, -649.6543) -> (51.9111, -657.7321) centre (60.2922, -650.18) cw
  arc A54 (-4.7601, -273.037) -> (-9.622, -270.5836) centre (-11.0781, -279.5132) ccw
  arc A55 (-59.6718, -354.8809) -> (-79.3222, -362.9588) centre (-70.9412, -355.4067) cw
  arc A56 (-95.1258, -348.4678) -> (-86.0885, -339.0761) centre (-84.8968, -349.2668) cw
  arc A57 (-72.8072, -333.1068) -> (-58.0221, -347.168) centre (-66.1625, -340.9237) cw
  arc A58 (-17.2817, -486.1862) -> (-8.472, -481.7418) centre (-19.9378, -469.9678) ccw
  arc A59 (120.553, -544.8551) -> (123.743, -544.5786) centre (120.0515, -520.5312) ccw
  arc A60 (111.5156, -554.2468) -> (120.553, -544.8551) centre (121.7446, -555.0458) cw
  arc A61 (-79.3222, -362.9588) -> (-80.1682, -362.0312) centre (-89.1467, -371.0704) ccw
  arc A62 (15.7364, -265.8867) -> (-3.9141, -273.9645) centre (4.4669, -266.4124) cw
  arc A63 (-19.7177, -259.4735) -> (-10.6804, -250.0818) centre (-9.4887, -260.2725) cw
  arc A64 (66.9361, -392.7476) -> (68.2176, -391.4992) centre (78.915, -403.7622) cw
  arc A65 (-19.4134, -506.9645) -> (-21.7533, -506.6116) centre (-18.481, -492.8491) cw
  arc A66 (45.899, -406.8602) -> (54.9363, -397.4685) centre (56.128, -407.6592) cw
  arc A67 (81.2094, -411.8194) -> (81.353, -413.2733) centre (62.2283, -414.4282) cw
  arc A68 (-21.7533, -506.6116) -> (-29.5091, -495.8545) centre (-19.2757, -496.6507) cw
  arc A69 (5.8013, -500.8137) -> (5.9449, -502.2676) centre (-13.1798, -503.4225) cw
  arc A70 (81.353, -413.2733) -> (61.7026, -421.3511) centre (70.0836, -413.799) cw
  arc A71 (73.2112, -641.9413) -> (71.418, -648.2004) centre (80.4428, -647.3996) ccw
  arc A72 (-85.0301, -359.5779) -> (-87.37, -359.2249) centre (-84.0977, -345.4624) cw
  arc A73 (146.9697, -560.66) -> (127.3193, -568.7378) centre (135.7003, -561.1857) cw
  arc A74 (-7.1905, -480.4935) -> (7.5945, -494.5547) centre (-0.5458, -488.3104) cw
  arc A75 (146.8261, -559.2061) -> (146.9697, -560.66) centre (127.845, -561.8148) cw
  arc A76 (17.386, -258.1737) -> (15.5928, -264.4328) centre (24.6176, -263.632) ccw
  arc A77 (-8.472, -481.7418) -> (-7.1905, -480.4935) centre (3.5069, -492.7565) cw
  arc A78 (36.1075, -643.2411) -> (45.1449, -633.8494) centre (46.3365, -644.0401) cw
  arc A79 (-82.8984, -338.7996) -> (-74.0887, -334.3552) centre (-85.5544, -322.5811) ccw
  arc A80 (55.9947, -417.9702) -> (53.6548, -417.6173) centre (56.9271, -403.8548) cw
  arc A81 (60.8566, -420.4236) -> (55.9947, -417.9702) centre (54.5386, -426.8999) ccw
  arc A82 (71.418, -648.2004) -> (71.5616, -649.6543) centre (52.4368, -650.8091) cw
  arc A83 (51.0651, -656.8045) -> (46.2032, -654.3512) centre (44.7471, -663.2808) ccw
  arc A84 (133.8343, -538.8858) -> (148.6193, -552.9471) centre (140.479, -546.7028) cw
  arc A85 (-80.1682, -362.0312) -> (-85.0301, -359.5779) centre (-86.4862, -368.5075) ccw
  arc A86 (132.5528, -540.1342) -> (133.8343, -538.8858) centre (144.5317, -551.1489) cw
  arc A87 (-13.7055, -510.3454) -> (-14.5516, -509.4179) centre (-23.53, -518.457) ccw
  arc A88 (-14.5516, -509.4179) -> (-19.4134, -506.9645) centre (-20.8696, -515.8942) ccw
  arc A89 (-74.0887, -334.3552) -> (-72.8072, -333.1068) centre (-62.1098, -345.3698) cw
  arc A90 (53.6548, -417.6173) -> (45.899, -406.8602) centre (56.1324, -407.6565) cw
  arc A91 (61.7026, -421.3511) -> (60.8566, -420.4236) centre (51.8781, -429.4628) ccw
  arc A92 (-59.8154, -353.4271) -> (-59.6718, -354.8809) centre (-78.7965, -356.0358) cw
  arc A93 (83.0027, -405.5604) -> (81.2094, -411.8194) centre (90.2342, -411.0187) ccw
  arc A94 (43.8633, -653.9982) -> (36.1075, -643.2411) centre (46.3409, -644.0374) cw
  arc A95 (68.2176, -391.4992) -> (83.0027, -405.5604) centre (74.8623, -399.3161) cw
  arc A96 (-29.5091, -495.8545) -> (-20.4718, -486.4628) centre (-19.2801, -496.6535) cw
  arc A97 (121.6114, -565.3569) -> (119.2714, -565.0039) centre (122.5438, -551.2415) cw
  arc A98 (126.4732, -567.8103) -> (121.6114, -565.3569) centre (120.1552, -574.2865) ccw
  arc A99 (-9.622, -270.5836) -> (-11.9619, -270.2306) centre (-8.6895, -256.4682) cw
  arc A100 (45.1449, -633.8494) -> (48.3349, -633.5729) centre (44.6434, -609.5255) ccw
  arc A101 (148.6193, -552.9471) -> (146.8261, -559.2061) centre (155.8509, -558.4053) ccw
  arc A102 (-7.4903, -249.8053) -> (1.3195, -245.3609) centre (-10.1463, -233.5868) ccw
  arc A103 (58.1264, -397.1919) -> (66.9361, -392.7476) centre (55.4703, -380.9735) ccw
  arc A104 (48.3349, -633.5729) -> (57.1447, -629.1285) centre (45.6789, -617.3544) ccw
  arc A105 (119.2714, -565.0039) -> (111.5156, -554.2468) centre (121.7491, -555.0431) cw
  arc A106 (7.5945, -494.5547) -> (5.8013, -500.8137) centre (14.8261, -500.013) ccw
  arc A107 (-20.4718, -486.4628) -> (-17.2817, -486.1862) centre (-20.9733, -462.1388) ccw
  arc A108 (-87.37, -359.2249) -> (-95.1258, -348.4678) centre (-84.8924, -349.2641) cw
  arc A109 (-49.8803, -118.5) -> (-69.5307, -126.5778) centre (-61.1497, -119.0257) cw
  arc A110 (-150.6468, -212.1912) -> (-152.9867, -211.8383) centre (-149.7143, -198.0758) cw
  arc A111 (-85.3344, -112.0869) -> (-76.297, -102.6952) centre (-75.1054, -112.8859) cw
  arc A112 (1.3195, -245.3609) -> (2.6009, -244.1125) centre (13.2983, -256.3756) cw
  arc A113 (-10.6804, -250.0818) -> (-7.4903, -249.8053) centre (-11.1819, -225.7579) ccw
  arc A114 (-152.9867, -211.8383) -> (-160.7425, -201.0812) centre (-150.5091, -201.8774) cw
  arc A115 (2.6009, -244.1125) -> (17.386, -258.1737) centre (9.2456, -251.9295) cw
  arc A116 (-160.7425, -201.0812) -> (-151.7051, -191.6894) centre (-150.5135, -201.8802) cw
  arc A117 (54.9363, -397.4685) -> (58.1264, -397.1919) centre (54.4348, -373.1445) ccw
  arc A118 (-64.2972, -97.9742) -> (-63.0157, -96.7259) centre (-52.3183, -108.9889) cw
  arc A119 (-63.0157, -96.7259) -> (-48.2307, -110.7871) centre (-56.371, -104.5428) cw
  arc A120 (-77.5786, -122.844) -> (-85.3344, -112.0869) centre (-75.1009, -112.8832) cw
  arc A121 (5.9449, -502.2676) -> (-13.7055, -510.3454) centre (-5.3245, -502.7933) cw
  arc A122 (-151.7051, -191.6894) -> (-148.5151, -191.4129) centre (-152.2066, -167.3655) ccw
  arc A123 (-69.5307, -126.5778) -> (-70.3768, -125.6503) centre (-79.3552, -134.6895) ccw
  arc A124 (-125.2884, -207.4943) -> (-144.9389, -215.5721) centre (-136.5578, -208.02) cw
  arc A125 (-125.432, -206.0404) -> (-125.2884, -207.4943) centre (-144.4132, -208.6492) cw
  arc A126 (-73.107, -102.4186) -> (-64.2972, -97.9742) centre (-75.763, -86.2002) ccw
  arc A127 (-139.7053, -186.9685) -> (-138.4238, -185.7202) centre (-127.7264, -197.9832) cw
  arc A128 (127.3193, -568.7378) -> (126.4732, -567.8103) centre (117.4948, -576.8494) ccw
  arc A129 (-58.0221, -347.168) -> (-59.8154, -353.4271) centre (-50.7905, -352.6263) ccw
  arc A130 (-138.4238, -185.7202) -> (-123.6388, -199.7814) centre (-131.7791, -193.5371) cw
  arc A131 (-123.6388, -199.7814) -> (-125.432, -206.0404) centre (-116.4072, -205.2397) ccw
  arc A132 (-145.7849, -214.6446) -> (-150.6468, -212.1912) centre (-152.1029, -221.1209) ccw
  arc A133 (-148.5151, -191.4129) -> (-139.7053, -186.9685) centre (-151.1711, -175.1945) ccw
  arc A134 (-86.0885, -339.0761) -> (-82.8984, -338.7996) centre (-86.59, -314.7522) ccw
  arc A135 (-144.9389, -215.5721) -> (-145.7849, -214.6446) centre (-154.7633, -223.6837) ccw
  arc A136 (-48.2307, -110.7871) -> (-50.0239, -117.0461) centre (-40.9991, -116.2454) ccw
  arc A137 (-75.2386, -123.1969) -> (-77.5786, -122.844) centre (-74.3062, -109.0815) cw
  arc A138 (57.1447, -629.1285) -> (58.4262, -627.8801) centre (69.1236, -640.1431) cw
  arc A139 (-50.0239, -117.0461) -> (-49.8803, -118.5) centre (-69.005, -119.6549) cw
  arc A140 (-76.297, -102.6952) -> (-73.107, -102.4186) centre (-76.7985, -78.3712) ccw
  arc A141 (46.2032, -654.3512) -> (43.8633, -653.9982) centre (47.1357, -640.2357) cw
  arc A142 (-3.9141, -273.9645) -> (-4.7601, -273.037) centre (-13.7386, -282.0761) ccw
  arc A143 (-70.3768, -125.6503) -> (-75.2386, -123.1969) centre (-76.6948, -132.1266) ccw
  arc A144 (89.7833, -401.0546) -> (97.6152, -423.5883) centre (93.0966, -412.531) cw
  arc A145 (37.6424, -656.2906) -> (31.3594, -642.8709) centre (46.3409, -644.0374) cw
  arc A146 (15.8916, -292.0741) -> (-6.6815, -293.4215) centre (4.3756, -288.9047) cw
  arc A147 (122.9961, -539.8749) -> (129.1496, -536.7999) centre (121.087, -528.3601) ccw
  arc A148 (129.1496, -536.7999) -> (130.7258, -535.2775) centre (144.5317, -551.1489) cw
  arc A149 (79.9919, -637.4356) -> (87.8237, -659.9693) centre (83.3051, -648.9119) cw
  arc A150 (54.6438, -392.71) -> (57.3795, -392.4883) centre (54.4348, -373.1445) ccw
  arc A151 (120.2605, -540.0967) -> (122.9961, -539.8749) centre (120.0515, -520.5312) ccw
  arc A152 (-27.9743, -508.904) -> (-34.2572, -495.4843) centre (-19.2757, -496.6507) cw
  arc A153 (6.1001, -528.455) -> (-16.473, -529.8025) centre (-5.4158, -525.2856) cw
  arc A154 (97.6152, -423.5883) -> (81.5082, -439.4607) centre (86.8596, -428.7825) cw
  arc A155 (-18.0287, -481.4826) -> (-11.8752, -478.4075) centre (-19.9378, -469.9678) ccw
  arc A156 (31.3594, -642.8709) -> (44.8524, -629.091) centre (46.3365, -644.0401) cw
  arc A157 (44.8524, -629.091) -> (47.588, -628.8692) centre (44.6434, -609.5255) ccw
  arc A158 (106.7676, -553.8766) -> (120.2605, -540.0967) centre (121.7446, -555.0458) cw
  arc A159 (55.3177, -624.2718) -> (79.9919, -637.4356) centre (65.0709, -635.6971) cw
  arc A160 (147.1249, -586.8474) -> (124.5518, -588.1948) centre (135.609, -583.678) cw
  arc A161 (113.0505, -567.2963) -> (106.7676, -553.8766) centre (121.7491, -555.0431) cw
  arc A162 (71.7168, -675.8417) -> (49.1437, -677.1891) centre (60.2008, -672.6723) cw
  arc A163 (87.8237, -659.9693) -> (71.7168, -675.8417) centre (77.0681, -665.1634) cw
  arc A164 (130.7258, -535.2775) -> (155.4, -548.4413) centre (140.479, -546.7028) cw
  arc A165 (47.588, -628.8692) -> (53.7415, -625.7942) centre (45.6789, -617.3544) ccw
  arc A166 (124.5518, -588.1948) -> (113.0505, -567.2963) centre (119.3568, -577.4398) cw
  arc A167 (53.7415, -625.7942) -> (55.3177, -624.2718) centre (69.1236, -640.1431) cw
  arc A168 (49.1437, -677.1891) -> (37.6424, -656.2906) centre (43.9487, -666.4341) cw
  arc A169 (-67.7004, -94.64) -> (-66.1242, -93.1176) centre (-52.3183, -108.9889) cw
  arc A170 (155.4, -548.4413) -> (163.2319, -570.975) centre (158.7132, -559.9176) cw
  arc A171 (-33.6181, -128.815) -> (-49.7251, -144.6874) centre (-44.3738, -134.0092) cw
  arc A172 (163.2319, -570.975) -> (147.1249, -586.8474) centre (152.4762, -576.1691) cw
  arc A173 (-77.4918, -331.0209) -> (-75.9156, -329.4985) centre (-62.1098, -345.3698) cw
  arc A174 (-151.9976, -186.931) -> (-149.262, -186.7093) centre (-152.2066, -167.3655) ccw
  arc A175 (-51.2415, -342.6623) -> (-43.4096, -365.196) centre (-47.9282, -354.1386) cw
  arc A176 (-24.4658, -259.1033) -> (-10.9728, -245.3234) centre (-9.4887, -260.2725) cw
  arc A177 (-8.2372, -245.1016) -> (-2.0837, -242.0266) centre (-10.1463, -233.5868) ccw
  arc A178 (-147.7063, -235.0292) -> (-159.2076, -214.1306) centre (-152.9013, -224.2741) cw
  arc A179 (-83.6453, -334.0959) -> (-77.4918, -331.0209) centre (-85.5544, -322.5811) ccw
  arc A180 (-75.9156, -329.4985) -> (-51.2415, -342.6623) centre (-66.1625, -340.9237) cw
  arc A181 (-99.8739, -348.0976) -> (-86.3809, -334.3177) centre (-84.8968, -349.2668) cw
  arc A182 (-59.5166, -381.0684) -> (-82.0896, -382.4158) centre (-71.0325, -377.899) cw
  arc A183 (-43.4096, -365.196) -> (-59.5166, -381.0684) centre (-54.1652, -370.3901) cw
  arc A184 (-82.0896, -382.4158) -> (-93.591, -361.5173) centre (-87.2847, -371.6608) cw
  arc A185 (-76.5895, -97.9367) -> (-73.8539, -97.715) centre (-76.7985, -78.3712) ccw
  arc A186 (-125.1332, -233.6817) -> (-147.7063, -235.0292) centre (-136.6492, -230.5123) cw
  arc A187 (-86.3809, -334.3177) -> (-83.6453, -334.0959) centre (-86.59, -314.7522) ccw
  arc A188 (-2.0837, -242.0266) -> (-0.5075, -240.5042) centre (13.2983, -256.3756) cw
  arc A189 (-73.8539, -97.715) -> (-67.7004, -94.64) centre (-75.763, -86.2002) ccw
  arc A190 (-93.591, -361.5173) -> (-99.8739, -348.0976) centre (-84.8924, -349.2641) cw
  arc A191 (24.1667, -253.668) -> (31.9985, -276.2017) centre (27.4799, -265.1443) cw
  arc A192 (-41.45, -106.2813) -> (-33.6181, -128.815) centre (-38.1368, -117.7577) cw
  arc A193 (-18.1828, -272.523) -> (-24.4658, -259.1033) centre (-9.4843, -260.2698) cw
  arc A194 (-66.1242, -93.1176) -> (-41.45, -106.2813) centre (-56.371, -104.5428) cw
  arc A195 (-49.7251, -144.6874) -> (-72.2982, -146.0349) centre (-61.241, -141.518) cw
  arc A196 (-10.9728, -245.3234) -> (-8.2372, -245.1016) centre (-11.1819, -225.7579) ccw
  arc A197 (-72.2982, -146.0349) -> (-83.7995, -125.1364) centre (-77.4932, -135.2798) cw
  arc A198 (-109.0263, -217.8093) -> (-125.1332, -233.6817) centre (-119.7819, -223.0034) cw
  arc A199 (-20.7643, -481.7043) -> (-18.0287, -481.4826) centre (-20.9733, -462.1388) ccw
  arc A200 (14.3752, -490.0489) -> (22.2071, -512.5826) centre (17.6884, -501.5252) cw
  arc A201 (-149.262, -186.7093) -> (-143.1085, -183.6342) centre (-151.1711, -175.1945) ccw
  arc A202 (58.9352, -440.8082) -> (47.4338, -419.9097) centre (53.7401, -430.0531) cw
  arc A203 (63.533, -389.4133) -> (65.1092, -387.8909) centre (78.915, -403.7622) cw
  arc A204 (81.5082, -439.4607) -> (58.9352, -440.8082) centre (69.9923, -436.2913) cw
  arc A205 (-143.1085, -183.6342) -> (-141.5323, -182.1119) centre (-127.7264, -197.9832) cw
  arc A206 (-165.4906, -200.711) -> (-151.9976, -186.931) centre (-150.5135, -201.8802) cw
  arc A207 (31.9985, -276.2017) -> (15.8916, -292.0741) centre (21.2429, -281.3958) cw
  arc A208 (65.1092, -387.8909) -> (89.7833, -401.0546) centre (74.8623, -399.3161) cw
  arc A209 (57.3795, -392.4883) -> (63.533, -389.4133) centre (55.4703, -380.9735) ccw
  arc A210 (22.2071, -512.5826) -> (6.1001, -528.455) centre (11.4514, -517.7768) cw
  arc A211 (-0.5075, -240.5042) -> (24.1667, -253.668) centre (9.2456, -251.9295) cw
  arc A212 (-34.2572, -495.4843) -> (-20.7643, -481.7043) centre (-19.2801, -496.6535) cw
  arc A213 (41.1509, -406.49) -> (54.6438, -392.71) centre (56.128, -407.6592) cw